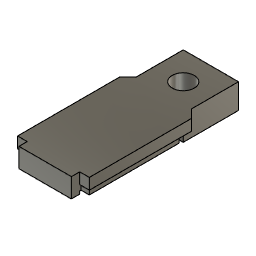
DTH11Holding (Autodesk Fusion 360 design; units mm, degrees)
Autodesk Fusion 360 part; units mm, degrees
sketch "Sketch1" plane through (0, 0, 0) normal (0, 0, 1) x (1, 0, 0)
  line L0 (0, 0) -> (10, 0)
  line L1 (10, 0) -> (10, 10)
  line L2 (10, 10) -> (0, 10)
  line L3 (0, 10) -> (0, 0)
  line L4 (0, 10) -> (10, 0)
  line L5 (0, 0) -> (10, 10)
  circle A0 centre (5, 5) radius 2
  dimension "d1" = 10
  dimension "d2" = 10
  dimension "d3" = 4
  constraint horizontal L0
  constraint vertical L1
  constraint horizontal L2
  constraint vertical L3
  constraint coincident L0.start L3.end
  constraint midpoint L5 A0.centre
  measures "d1" distance of L0.start L0.end
  measures "d2" distance of L0.start L2.end
  measures "d3" diameter of A0
extrude "Extrude1" add sketch "Sketch1" along normal blind 2.5 contours L0 L4 L5 A0 | L3 L4 L5 A0 | L1 L4 L5 A0 | L2 L4 L5 A0
sketch "Sketch2" plane through (0, 0, 2.5) normal (0, 0, 1) x (-1, 0, 0)
  circle A0 centre (-5, -5) radius 2
  line L0 (0, -10) -> (0, 0)
  line L1 (0, 0) -> (-10, 0)
  line L2 (-10, 0) -> (-10, -10)
  line L3 (-10, -10) -> (0, -10)
  line L4 (0, 0) -> (-10, 0)
  line L5 (-10, 0) -> (-10, 2)
  line L6 (-10, 2) -> (0, 2)
  line L7 (0, 2) -> (0, 0)
  line L8 (0, 0) -> (-10, 0)
  line L9 (-10, 0) -> (-10, 1.5)
  line L10 (-10, 1.5) -> (0, 1.5)
  line L11 (0, 1.5) -> (0, 0)
  line L12 (-5, 0) -> (3, 0)
  line L13 (3, 0) -> (3, 1.5)
  line L14 (3, 1.5) -> (-5, 1.5)
  line L15 (-5, 1.5) -> (-5, 0)
  line L16 (-5, 0) -> (-13, 0)
  line L17 (-13, 0) -> (-13, 1.5)
  line L18 (-13, 1.5) -> (-5, 1.5)
  line L19 (-5, 1.5) -> (-5, 0)
  line L20 (3, 0) -> (1.5, 0)
  line L21 (1.5, 0) -> (1.5, 1.5)
  line L22 (1.5, 1.5) -> (3, 1.5)
  line L23 (3, 1.5) -> (3, 0)
  line L24 (3, 0) -> (1.5, 0)
  line L25 (1.5, 0) -> (1.5, 20)
  line L26 (1.5, 20) -> (3, 20)
  line L27 (3, 20) -> (3, 0)
  line L28 (-13, 0) -> (-11.5, 0)
  line L29 (-11.5, 0) -> (-11.5, 20)
  line L30 (-11.5, 20) -> (-13, 20)
  line L31 (-13, 20) -> (-13, 0)
  line L32 (1.5, 20) -> (0, 20)
  line L33 (0, 20) -> (0, 18.5)
  line L34 (0, 18.5) -> (1.5, 18.5)
  line L35 (1.5, 18.5) -> (1.5, 20)
  line L36 (-11.5, 20) -> (-10, 20)
  line L37 (-10, 20) -> (-10, 18.5)
  line L38 (-10, 18.5) -> (-11.5, 18.5)
  line L39 (-11.5, 18.5) -> (-11.5, 20)
  line L40 (1.5, 2) -> (-11.5, 2)
  line L41 (-11.5, 2) -> (-11.5, 18.5)
  line L42 (-11.5, 18.5) -> (1.5, 18.5)
  line L43 (1.5, 18.5) -> (1.5, 2)
  line L44 (1.5, 0) -> (0, -1.5)
  line L45 (1.5, 0) -> (3.6213, 0) construction
  line L46 (-11.5, 0) -> (-10, -1.5)
  dimension "d6" = 2
  dimension "d7" = 1.5
  dimension "d8" = 8
  dimension "d9" = 20
  dimension "d10" = 1.5
  dimension "d11" = 20
  dimension "d12" = 1.5
  dimension "d13" = 1.5
  dimension "d14" = 1.5
  dimension "d15" = 1.5
  dimension "d16" = 135
  dimension "d17" = 90
  constraint horizontal L4
  constraint vertical L5
  constraint horizontal L6
  constraint vertical L7
  constraint coincident L0.end L1.start
  constraint horizontal L8
  constraint vertical L9
  constraint horizontal L10
  constraint vertical L11
  constraint horizontal L12
  constraint vertical L13
  constraint horizontal L14
  constraint vertical L15
  constraint midpoint L4 L12.start
  constraint horizontal L16
  constraint vertical L17
  constraint horizontal L18
  constraint vertical L19
  constraint horizontal L20
  constraint vertical L21
  constraint horizontal L22
  constraint vertical L23
  constraint coincident L14 L21.end
  constraint horizontal L24
  constraint vertical L25
  constraint horizontal L26
  constraint vertical L27
  constraint horizontal L28
  constraint vertical L29
  constraint horizontal L30
  constraint vertical L31
  constraint horizontal L32
  constraint vertical L33
  constraint horizontal L34
  constraint vertical L35
  constraint horizontal L36
  constraint vertical L37
  constraint horizontal L38
  constraint vertical L39
  constraint horizontal L40
  constraint vertical L41
  constraint horizontal L42
  constraint vertical L43
  constraint horizontal L45
  constraint coincident L0 L44.end
  constraint coincident L2 L46.end
  measures "d6" distance of L0.end L6.end
  measures "d7" distance of L0.end L10.end
  measures "d8" distance of L12.start L12.end
  measures "d9" distance of L12.end L26.end
  measures "d10" distance of L16.end L28.end
  measures "d11" distance of L16.end L30.end
  measures "d12" distance of L25.end L32.end
  measures "d13" distance of L25.end L34.end
  measures "d14" distance of L29.end L36.end
  measures "d15" distance of L29.end L38.end
  measures "d16" angle of L44 L45
  measures "d17" angle of L44 L46
extrude "Extrude2" add sketch "Sketch2" along normal blind 2 contours L0 L1 L2 L3 L4 L8 L12 L16 | L0 L12 L44 | L1 L4 L7 L8 L10 L11 L12 L14 L15 L19 | L7 L11 L12 L14 L21 L25 | L2 L16 L46 | L1 L4 L5 L8 L9 L10 L15 L16 L18 L19 | L5 L6 L7 L10 L14 L18 L40 | L7 L14 L25 L40 | L5 L9 L16 L18 L29 | L6 L25 L29 L34 L38 L40 L41 L42 L43 | L5 L18 L29 L40
sketch "Sketch3" plane through (0, 0, 2.5) normal (0, 0, -1) x (1, 0, 0)
  line L0 (10, 0) -> (10, -1.5)
  line L1 (10, -1.5) -> (11.5, 0)
  line L2 (11.5, 0) -> (11.5, 18.5)
  line L3 (11.5, 18.5) -> (-1.5, 18.5)
  line L4 (-1.5, 18.5) -> (-1.5, 0)
  line L5 (-1.5, 0) -> (0, -1.5)
  line L6 (0, -1.5) -> (0, 0)
  line L7 (0, 0) -> (10, 0)
  line L8 (-1.5, 0) -> (11.5, 0)
  line L9 (11.5, 0) -> (11.5, -1.5)
  line L10 (11.5, -1.5) -> (-1.5, -1.5)
  line L11 (-1.5, -1.5) -> (-1.5, 0)
  line L12 (-1.5, 0) -> (11.5, 0)
  line L13 (11.5, 0) -> (11.5, 2)
  line L14 (11.5, 2) -> (-1.5, 2)
  line L15 (-1.5, 2) -> (-1.5, 0)
  line L16 (-1.5, 18.5) -> (-1, 18.5)
  line L17 (-1, 2) -> (-1.5, 2)
  line L18 (-1.5, 2) -> (-1.5, 18.5)
  line L19 (11.5, 18.5) -> (11, 18.5)
  line L20 (11, 2) -> (11.5, 2)
  line L21 (11.5, 2) -> (11.5, 18.5)
  line L22 (-1.5, 18.5) -> (0, 18.5)
  line L23 (0, 18.5) -> (0, 20)
  line L24 (0, 20) -> (-1.5, 20)
  line L25 (-1.5, 20) -> (-1.5, 18.5)
  line L26 (11.5, 18.5) -> (10, 18.5)
  line L27 (10, 18.5) -> (10, 20)
  line L28 (10, 20) -> (11.5, 20)
  line L29 (11.5, 20) -> (11.5, 18.5)
  line L30 (10, 20) -> (9.75, 20)
  line L31 (9.75, 20) -> (9.75, 18.5)
  line L32 (9.75, 18.5) -> (10, 18.5)
  line L33 (10, 18.5) -> (10, 20)
  line L34 (0, 20) -> (0.25, 20)
  line L35 (0.25, 20) -> (0.25, 18.5)
  line L36 (0.25, 18.5) -> (0, 18.5)
  line L37 (0, 18.5) -> (0, 20)
  line L38 (-1.5, 20) -> (-1.25, 20)
  line L39 (-1.25, 20) -> (-1.25, 2)
  line L40 (-1.25, 2) -> (-1.5, 2)
  line L41 (-1.5, 2) -> (-1.5, 20)
  line L42 (11.5, 2) -> (11.25, 2)
  line L43 (11.25, 2) -> (11.25, 18.5)
  line L44 (11.25, 18.5) -> (11.5, 18.5)
  line L45 (11.5, 18.5) -> (11.5, 2)
  line L46 (-1.5, 18.5) -> (0.25, 18.5)
  line L47 (0.25, 18.5) -> (0.25, 18.25)
  line L48 (0.25, 18.25) -> (-1.5, 18.25)
  line L49 (-1.5, 18.25) -> (-1.5, 18.5)
  line L50 (9.75, 18.5) -> (11.25, 18.5)
  line L51 (11.25, 18.5) -> (11.25, 18.25)
  line L52 (11.25, 18.25) -> (9.75, 18.25)
  line L53 (9.75, 18.25) -> (9.75, 18.5)
  line L54 (0.25, 20) -> (9.75, 20)
  line L55 (9.75, 20) -> (9.75, 18.5)
  line L56 (9.75, 18.5) -> (0.25, 18.5)
  line L57 (0.25, 18.5) -> (0.25, 20)
  dimension "d20" = 13
  dimension "d21" = 2
  dimension "d22" = 0.5
  dimension "d23" = 0.5
  dimension "d24" = 1.5
  dimension "d25" = 1.5
  dimension "d26" = 1.5
  dimension "d27" = 1.5
  dimension "d28" = 0.25
  dimension "d29" = 0.25
  dimension "d30" = 0.25
  dimension "d31" = 0.25
  dimension "d32" = 0.25
  dimension "d33" = 0.25
  constraint horizontal L8
  constraint vertical L9
  constraint horizontal L10
  constraint vertical L11
  constraint coincident L4.end L5.start
  constraint horizontal L12
  constraint vertical L13
  constraint horizontal L14
  constraint vertical L15
  constraint horizontal L16
  constraint horizontal L17
  constraint vertical L18
  constraint coincident L3.end L4.start
  constraint horizontal L19
  constraint horizontal L20
  constraint vertical L21
  constraint coincident L2.end L3.start
  constraint horizontal L22
  constraint vertical L23
  constraint horizontal L24
  constraint vertical L25
  constraint horizontal L26
  constraint vertical L27
  constraint horizontal L28
  constraint vertical L29
  constraint horizontal L30
  constraint vertical L31
  constraint horizontal L32
  constraint vertical L33
  constraint coincident L3 L31.end
  constraint horizontal L34
  constraint vertical L35
  constraint horizontal L36
  constraint vertical L37
  constraint coincident L3 L35.end
  constraint horizontal L38
  constraint vertical L39
  constraint horizontal L40
  constraint vertical L41
  constraint horizontal L42
  constraint vertical L43
  constraint horizontal L44
  constraint vertical L45
  constraint horizontal L46
  constraint vertical L47
  constraint horizontal L48
  constraint vertical L49
  constraint horizontal L50
  constraint vertical L51
  constraint horizontal L52
  constraint vertical L53
  constraint horizontal L54
  constraint vertical L55
  constraint horizontal L56
  constraint vertical L57
  measures "d20" distance of L4.end L1.end
  measures "d21" distance of L4.end L14.end
  measures "d22" distance of L3.end L16.end
  measures "d23" distance of L2.end L19.end
  measures "d24" distance of L3.end L22.end
  measures "d25" distance of L3.end L24.end
  measures "d26" distance of L2.end L26.end
  measures "d27" distance of L2.end L28.end
  measures "d28" distance of L27.end L30.end
  measures "d29" distance of L23.end L34.end
  measures "d30" distance of L24.end L38.end
  measures "d31" distance of L13.end L42.end
  measures "d32" distance of L3.end L48.end
  measures "d33" distance of L31.end L52.end
extrude "Extrude3" add sketch "Sketch3" along normal blind 1 contours L3 L14 L17 L20 L39 L43 L47 L48 L52 L53 L56 | L3 L31 L35 L54 L55 L56 L57
sketch "Sketch4" plane through (0, 0, 1.5) normal (0, 0, -1) x (1, 0, 0)
  line L0 (0.25, 18.25) -> (-1.25, 18.25)
  line L1 (-1.25, 18.25) -> (-1.25, 2)
  line L2 (-1.25, 2) -> (11.25, 2)
  line L3 (11.25, 2) -> (11.25, 18.25)
  line L4 (11.25, 18.25) -> (9.75, 18.25)
  line L5 (9.75, 18.25) -> (9.75, 20)
  line L6 (9.75, 20) -> (0.25, 20)
  line L7 (0.25, 20) -> (0.25, 18.25)
  line L8 (0.25, 20) -> (9.75, 20)
  line L9 (9.75, 20) -> (9.75, 18.5)
  line L10 (9.75, 18.5) -> (0.25, 18.5)
  line L11 (0.25, 18.5) -> (0.25, 20)
  dimension "d36" = 1.5
  constraint horizontal L8
  constraint vertical L9
  constraint horizontal L10
  constraint vertical L11
  constraint coincident L6.end L7.start
  measures "d36" distance of L6.end L10.end
extrude "Extrude4" add sketch "Sketch4" along normal blind 0.5 contours L5 L6 L7 L8 L9 L10 L11
extrude "Extrude5" add 1 faces at (3.4167, -19, 2.5) along direction (0, 0, 1) blind 2
